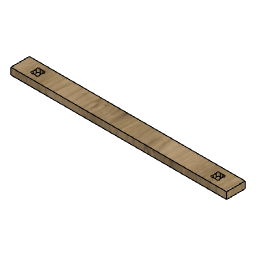
seta (Autodesk Fusion 360 design; units mm, degrees)
Autodesk Fusion 360 part; units mm, degrees
sketch "Sketch1" plane through (0, 0, 0) normal (0, 0, 1) x (1, 0, 0)
  line L0 (0, 0) -> (580, 0)
  line L1 (580, 0) -> (580, 50)
  line L2 (580, 50) -> (0, 50)
  line L3 (0, 50) -> (0, 0)
  dimension "d5" = 580
  dimension "d6" = 50
  constraint horizontal L0
  constraint vertical L1
  constraint horizontal L2
  constraint vertical L3
  constraint coincident L0.start L3.end
  measures "d5" distance of L0.start L0.end
  measures "d6" distance of L0.start L2.end
extrude "Extrude1" add sketch "Sketch1" along normal blind 18
sketch "Sketch2" plane through (0, 0, 18) normal (0, 0, 1) x (-1, 0, 0)
  line L0 (0, -50) -> (0, 0)
  line L1 (0, 0) -> (-580, 0)
  line L2 (-580, 0) -> (-580, -50)
  line L3 (-580, -50) -> (0, -50)
  line L4 (-44.3517, -35) -> (-51.6483, -35)
  line L5 (-57, -29.0536) -> (-57, -20.9464)
  line L6 (-51.6483, -15) -> (-44.3517, -15)
  line L7 (-39, -20.9464) -> (-39, -29.0536)
  line L8 (-44.3517, -35) -> (-51.6483, -35)
  line L9 (-57, -29.0536) -> (-57, -20.9464)
  line L10 (-51.6483, -15) -> (-44.3517, -15)
  line L11 (-39, -20.9464) -> (-39, -29.0536)
  line L12 (-44.3517, -35) -> (-51.6483, -35)
  line L13 (-57, -29.0536) -> (-57, -20.9464)
  line L14 (-51.6483, -15) -> (-44.3517, -15)
  line L15 (-39, -20.9464) -> (-39, -29.0536)
  line L16 (-528.3517, -35) -> (-535.6483, -35)
  line L17 (-541, -29.0536) -> (-541, -20.9464)
  line L18 (-535.6483, -15) -> (-528.3517, -15)
  line L19 (-523, -20.9464) -> (-523, -29.0536)
  arc A0 (-44.3517, -35) -> (-39, -29.0536) centre (-41.6759, -32.0268) ccw
  arc A1 (-44.3517, -35) -> (-39, -29.0536) centre (-41.6759, -32.0268) ccw
  arc A2 (-44.3517, -35) -> (-39, -29.0536) centre (-41.6759, -32.0268) ccw
  arc A3 (-57, -29.0536) -> (-51.6483, -35) centre (-54.3241, -32.0268) ccw
  arc A4 (-57, -29.0536) -> (-51.6483, -35) centre (-54.3241, -32.0268) ccw
  arc A5 (-57, -29.0536) -> (-51.6483, -35) centre (-54.3241, -32.0268) ccw
  arc A6 (-51.6483, -15) -> (-57, -20.9464) centre (-54.3241, -17.9732) ccw
  arc A7 (-51.6483, -15) -> (-57, -20.9464) centre (-54.3241, -17.9732) ccw
  arc A8 (-51.6483, -15) -> (-57, -20.9464) centre (-54.3241, -17.9732) ccw
  arc A9 (-39, -20.9464) -> (-44.3517, -15) centre (-41.6759, -17.9732) ccw
  arc A10 (-39, -20.9464) -> (-44.3517, -15) centre (-41.6759, -17.9732) ccw
  arc A11 (-39, -20.9464) -> (-44.3517, -15) centre (-41.6759, -17.9732) ccw
  arc A12 (-528.3517, -35) -> (-523, -29.0536) centre (-525.6759, -32.0268) ccw
  arc A13 (-523, -20.9464) -> (-528.3517, -15) centre (-525.6759, -17.9732) ccw
  arc A14 (-535.6483, -15) -> (-541, -20.9464) centre (-538.3241, -17.9732) ccw
  arc A15 (-541, -29.0536) -> (-535.6483, -35) centre (-538.3241, -32.0268) ccw
  dimension "d13" = 8
  dimension "d14" = 8
  dimension "d15" = 8
  dimension "d16" = 8
  dimension "d19" = 8
  dimension "d20" = 8
  dimension "d21" = 8
  dimension "d22" = 8
  dimension "d25" = 8
  dimension "d26" = 8
  dimension "d27" = 8
  dimension "d28" = 8
  dimension "d31" = 8
  dimension "d32" = 8
  dimension "d33" = 8
  dimension "d34" = 8
  constraint horizontal L4
  constraint vertical L5
  constraint horizontal L6
  constraint vertical L7
  constraint horizontal L8
  constraint vertical L9
  constraint horizontal L10
  constraint vertical L11
  constraint horizontal L12
  constraint vertical L13
  constraint horizontal L14
  constraint vertical L15
  constraint horizontal L16
  constraint vertical L17
  constraint horizontal L18
  constraint vertical L19
  measures "d13" diameter of A2
  measures "d14" diameter of A5
  measures "d15" diameter of A10
  measures "d16" diameter of A8
  measures "d19" diameter of A0
  measures "d20" diameter of A4
  measures "d21" diameter of A11
  measures "d22" diameter of A6
  measures "d25" diameter of A1
  measures "d26" diameter of A3
  measures "d27" diameter of A9
  measures "d28" diameter of A7
  measures "d31" diameter of A12
  measures "d32" diameter of A15
  measures "d33" diameter of A13
  measures "d34" diameter of A14
extrude "Extrude2" cut sketch "Sketch2" against normal blind 10 contours L4 L5 L6 L7 L8 L9 L10 L11 L12 L13 L14 L15 A0 A1 A2 A3 A4 A5 A6 A7 A8 A9 A10 A11 | L16 L17 L18 L19 A12 A13 A14 A15
equation "breidd_seta = 50 mm"
equation "lengd_seta = 580 mm"
equation "t_seta = 18 mm"
equation "dog_r = 8 mm"
equation "d5 = lengd_seta"
equation "d6 = breidd_seta"
equation "d7 = t_seta"
equation "d13 = dog_r"
equation "d14 = dog_r"
equation "d15 = dog_r"
equation "d16 = dog_r"
equation "d19 = dog_r"
equation "d20 = dog_r"
equation "d21 = dog_r"
equation "d22 = dog_r"
equation "d25 = dog_r"
equation "d26 = dog_r"
equation "d27 = dog_r"
equation "d28 = dog_r"
equation "d31 = dog_r"
equation "d32 = dog_r"
equation "d33 = dog_r"
equation "d34 = dog_r"
